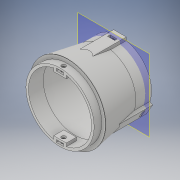
# Autodesk Inventor part: endkappen_V3
Saved by Autodesk Inventor 2017 (Build 210142000, 142)
## iProperties
Part Number: endkappen_V3
Material: Generisch
Document SubType Name: Modeling
Designer: Fabio
Density: 1 g/cm^3
Appearance: Vorgabe
Author: Fabio
Autodesk Inventor part; units mm, degrees
ref_plane "YZ Plane" through (0, 0, 0) normal (1, 0, 0) x (0, 1, 0)
ref_plane "XZ Plane" through (0, 0, 0) normal (0, 1, 0) x (-1, 0, 0)
ref_plane "XY Plane" through (0, 0, 0) normal (0, 0, 1) x (1, 0, 0)
sketch "Skizze2" plane through (0, 0, 0) normal (1, 0, 0) x (0, 1, 0)
  line L0 (0, 0) -> (48.6481, 0)
  line L1 (47.4748, 20) -> (47.4748, 25)
  line L2 (6, 30) -> (6, 27)
  line L3 (6, 27) -> (0, 27)
  line L4 (6.2626, 30) -> (6, 30)
  line L5 (11.7576, 25) -> (0, 25)
  line L6 (0, 25) -> (0, 27)
  line L7 (0, 0) -> (0, 25) construction
  line L8 (40.5337, 20) -> (47.4748, 20)
  line L9 (11.7576, 25) -> (40.5337, 20)
  line L10 (47.4748, 25) -> (35.0388, 25)
  line L11 (6.2626, 30) -> (35.0388, 25)
  dimension "d164" = 60
  dimension "d166" = 54
  dimension "d167" = 50
  dimension "d168" = 6
  dimension "d171" = 47.4748
  dimension "d174" = 40.5337
  dimension "d203" = 3
  dimension "d204" = 40
  dimension "d205" = 5
  dimension "d206" = 170.143
  dimension "d207" = 12.436
  constraints: 24 end point, 5 horizontal, 2 vertical, 1 parallel, 1 perpendicular
  measures "d164" diameter of L4 L0
  measures "d166" diameter of L3 L0
  measures "d167" diameter of L5 L0
  measures "d168" distance of L2.end L3.end
  measures "d171" distance of L5.end L1.end
  measures "d174" distance from line of L7 L8.start
  measures "d203" distance of L2.start L2.end
  measures "d204" diameter of L8 L0
  measures "d205" distance of L1.start L1.end
  measures "d206" angle of L5 L9
  measures "d207" distance of L1.end L10.end
revolve "Umdrehung1" add sketch "Skizze2" angle 360 about axis through (0, 0, 0) along (0, 1, 0)
sketch "Skizze18" plane through (0, 0, 0) normal (0, -1, 0) x (1, 0, 0)
  circle A0 centre (0, 0) radius 25 projected
  line L0 (5, -22) -> (-5, -22)
  line L1 (-5, -22) -> (-5, -25)
  line L2 (-5, -25) -> (5, -25)
  line L3 (5, -25) -> (5, -22)
  line L4 (5, -22) -> (-5, -25) construction
  line L5 (-5, -22) -> (5, -25) construction
  line L6 (0, -23.5) -> (0, 0) construction
  line L7 (0, 0) -> (9.0804, 0) construction
  line L8 (5, 22) -> (-5, 22)
  line L9 (-5, 22) -> (-5, 25)
  line L10 (-5, 25) -> (5, 25)
  line L11 (5, 25) -> (5, 22)
  dimension "d176" = 10
  dimension "d177" = 3
  dimension "d178" = 22
  constraints: 24 end point, 4 symmetric about line, 2 horizontal, 2 midpoint, 2 parallel, 1 perpendicular, 1 vertical
  measures "d176" distance of L2.end L1.end
  measures "d177" distance of L0.end L1.end
  measures "d178" distance from line of point (0, 0) L0
extrude "Extrusion14" add sketch "Skizze18" against normal blind 8 contours L11 L8 L9 A0 | A0 L10 L11 | L3 L2 A0 | A0 L1 L0 L3 | A0 L9 L10 | L2 L1 A0
sketch "Skizze19" plane through (0, 0, 0) normal (0, -1, 0) x (1, 0, 0)
  arc A0 (-5, -24.4949) -> (5, -24.4949) centre (0, 0) ccw projected
  line L0 (0, 0) -> (9.7237, 0) construction
  line L1 (0, -24.5) -> (0, 0) construction
  line L2 (2.85, -23.5) -> (-2.85, -23.5)
  line L3 (-2.85, -23.5) -> (-2.85, -25.5)
  line L4 (-2.85, -25.5) -> (2.85, -25.5)
  line L5 (2.85, -25.5) -> (2.85, -23.5)
  line L6 (2.85, -23.5) -> (-2.85, -25.5) construction
  line L7 (-2.85, -23.5) -> (2.85, -25.5) construction
  line L8 (2.85, 23.5) -> (-2.85, 23.5)
  line L9 (-2.85, 23.5) -> (-2.85, 25.5)
  line L10 (-2.85, 25.5) -> (2.85, 25.5)
  line L11 (2.85, 25.5) -> (2.85, 23.5)
  dimension "d236" = 5.7
  dimension "d237" = 2
  dimension "d238" = 23.5
  constraints: 24 end point, 4 symmetric about line, 2 horizontal, 2 midpoint, 2 parallel, 1 perpendicular, 1 vertical
  measures "d236" distance of L4.end L3.end
  measures "d237" distance of L3.end L2.end
  measures "d238" distance between parallel lines of L0 L2
extrude "Extrusion15" cut sketch "Skizze19" against normal blind 5.7
sketch "Skizze20" plane through (5, 0, 22) normal (0, 0, -1) x (-1, 0, 0)
  line L0 (10, 0) -> (0, 0) projected
  line L1 (10, 0) -> (10, 8) projected
  point P0 (5, 0)
  point P1 (5, 2.85)
  dimension "d185" = 2.85
  dimension "d186" = 5
  measures "d185" distance from line of L0 point (5, 2.85)
  measures "d186" distance from line of L1 point (5, 2.85)
hole "Bohrung4" at (0, 2.85, 22) direction (0, 0, 1) diameter 3.3 end through all
sketch "Skizze21" plane through (-5, 0, -22) normal (0, 0, 1) x (1, 0, 0)
  line L0 (10, 0) -> (0, 0) projected
  line L1 (0, 0) -> (0, 8) projected
  point P0 (5, 0)
  point P1 (5, 2.85)
  dimension "d194" = 2.85
  dimension "d195" = 5
  measures "d194" distance from line of point (5, 2.85) L0
  measures "d195" distance from line of L1 point (5, 2.85)
hole "Bohrung5" at (0, 2.85, -22) direction (0, 0, -1) diameter 3.3 end through all
sketch "Skizze22" plane through (0, 47.4748, 0) normal (0, 1, 0) x (1, 0, 0)
  circle A0 centre (0, 0) radius 25 projected
  line L0 (-5, -27) -> (5, -27)
  line L1 (5, -27) -> (5, -23)
  line L2 (5, -23) -> (-5, -23)
  line L3 (-5, -23) -> (-5, -27)
  arc A1 (-5, -24.4949) -> (5, -24.4949) centre (0, 0) ccw projected
  line L4 (-5, -27) -> (5, -23) construction
  line L5 (5, -27) -> (-5, -23) construction
  line L6 (0, -25) -> (0, 0) construction
  line L7 (25.8827, 9.1699) -> (20.8827, 17.8301)
  line L8 (22.4186, 7.1699) -> (25.8827, 9.1699)
  line L9 (17.4186, 15.8301) -> (22.4186, 7.1699)
  line L10 (20.8827, 17.8301) -> (17.4186, 15.8301)
  line L11 (-20.8827, 17.8301) -> (-25.8827, 9.1699)
  line L12 (-17.4186, 15.8301) -> (-20.8827, 17.8301)
  line L13 (-22.4186, 7.1699) -> (-17.4186, 15.8301)
  line L14 (-25.8827, 9.1699) -> (-22.4186, 7.1699)
  dimension "d208" = 10
  dimension "d209" = 4
  dimension "d212" = 360
  constraints: 30 end point, 2 midpoint, 2 parallel, 2 point on circle, 1 horizontal, 1 perpendicular, 1 vertical, 25 other
  measures "d208" distance of L2.end L1.end
  measures "d209" distance of L1.end L0.end
extrude "Extrusion16" add sketch "Skizze22" against normal blind 30 contours L3 L2 L1 A0 | A0 L1 L0 L3 | L14 L11 L12 A0 | A0 L12 L13 L14 | L8 L9 L10 A0 | A0 L10 L7 L8
delete faces "Fläche löschen8" heal yes whole lump no faces at (-19.3891, 18.9869, -12.4171) (-20.4718, 17.4748, -11.1737)
delete faces "Fläche löschen9" heal yes whole lump no faces at (1.1063, 18.9488, 23) (-0.5592, 17.4748, 23.316)
delete faces "Fläche löschen10" heal yes whole lump no faces at (20.4718, 17.4748, -11.1737) (20.4481, 18.9869, -10.5829)
ref_plane "Arbeitsebene3" through (-5, 42.4748, 27) normal (0, 1, 0) x (1, 0, 0)
sketch "Skizze23" plane through (-5, 42.4748, 27) normal (0, 1, 0) x (1, 0, 0)
  circle A0 centre (5, 27) radius 25 projected
  line L0 (5, 27) -> (5, -9.3664) construction
  line L1 (0, 0) -> (10, 0) construction
  line L2 (2.15, -5.7) -> (7.85, -5.7)
  line L3 (7.85, -5.7) -> (7.85, 5.7)
  line L4 (7.85, 5.7) -> (2.15, 5.7)
  line L5 (2.15, 5.7) -> (2.15, -5.7)
  line L6 (2.15, -5.7) -> (7.85, 5.7) construction
  line L7 (7.85, -5.7) -> (2.15, 5.7) construction
  line L8 (22.0213, 40.1182) -> (24.8713, 35.1818)
  line L9 (31.894, 45.8182) -> (22.0213, 40.1182)
  line L10 (24.8713, 35.1818) -> (34.744, 40.8818)
  line L11 (34.744, 40.8818) -> (31.894, 45.8182)
  line L12 (-14.8713, 35.1818) -> (-12.0213, 40.1182)
  line L13 (-24.744, 40.8818) -> (-14.8713, 35.1818)
  line L14 (-12.0213, 40.1182) -> (-21.894, 45.8182)
  line L15 (-21.894, 45.8182) -> (-24.744, 40.8818)
  point P0 (5, 0)
  dimension "d217" = 5.7
  dimension "d218" = 11.4
  dimension "d221" = 360
  constraints: 30 end point, 3 midpoint, 2 parallel, 1 horizontal, 1 perpendicular, 1 vertical, 25 other
  measures "d217" distance of L4.end L3.end
  measures "d218" distance of L3.end L2.end
extrude "Extrusion17" cut sketch "Skizze23" against normal blind 2 contours L10 L8 L9 A0 | A0 L9 L11 L10 | L3 L2 L5 A0 | A0 L5 L4 L3 | L14 L12 L13 A0 | A0 L13 L15 L14
sketch "Skizze24" plane through (-5, 47.4748, 27) normal (0, 1, 0) x (1, 0, 0)
  line L0 (7.85, 0) -> (2.15, 0) projected
  line L1 (7.85, 5.7) -> (7.85, 0) projected
  line L2 (2.15, 5.7) -> (7.85, 5.7) projected
  line L3 (2.15, 0) -> (2.15, 5.7) projected
  line L4 (2.15, 5.7) -> (7.85, 0) construction
  line L5 (7.85, 5.7) -> (2.15, 0) construction
  point P0 (5, 27)
  point P1 (5, 2.85)
  point P2 (25.9145, 39.075)
  point P3 (-15.9145, 39.075)
  dimension "d227" = 360
  constraints: 4 end point, 1 midpoint, 1 perpendicular, 4 other
hole "Bohrung6" at (0, 47.4748, 24.15) at (20.9145, 47.4748, -12.075) at (-20.9145, 47.4748, -12.075) direction (0, -1, 0) diameter 3.3 depth 15 tip angle 118
